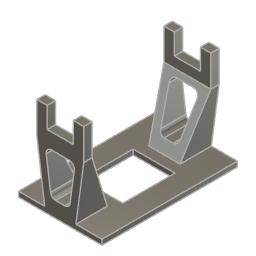
jack_stands_R (Autodesk Fusion 360 design; units mm, degrees)
Autodesk Fusion 360 part; units mm, degrees
note: some values were not read from the file. Set by a fixed rule: which sketch regions a step uses.
sketch "Esquisse1" plane through (0, 0, 0) normal (0, 0, 1) x (1, 0, 0)
  line L0 (27.5, 70) -> (52.5, 70)
  line L1 (52.5, 70) -> (52.5, 90)
  line L2 (27.5, 70) -> (27.5, 90)
  line L3 (27.5, 90) -> (17.5, 90)
  line L4 (52.5, 90) -> (62.5, 90)
  line L5 (62.5, 90) -> (62.5, 60)
  line L6 (17.5, 90) -> (17.5, 60)
  line L7 (17.5, 60) -> (25, 5)
  line L8 (25, 5) -> (0, 5)
  line L9 (0, 5) -> (0, 0)
  line L10 (0, 0) -> (80, 0)
  line L11 (80, 0) -> (80, 5)
  line L12 (80, 5) -> (55, 5)
  line L13 (55, 5) -> (62.5, 60)
  dimension "d1" = 70
  dimension "d2" = 25
  dimension "d3" = 20
  dimension "d4" = 10
  dimension "d5" = 30
  dimension "d8" = 5
  dimension "d10" = 10
  dimension "d27" = 80
  dimension "d28" = 45
  dimension "d29" = 17.5
  dimension "d30" = 30
  constraint horizontal L0
  constraint perpendicular L0 L1
  constraint perpendicular L0 L2
  constraint perpendicular L2 L3
  constraint perpendicular L1 L4
  constraint perpendicular L4 L5
  constraint equal L3 L4
  constraint perpendicular L3 L6
  constraint perpendicular L6 L8
  constraint coincident L9.end L10.start
  constraint perpendicular L8 L9
  constraint perpendicular L9 L10
  constraint perpendicular L10 L11
  constraint perpendicular L9 L12
  constraint horizontal L5.end L6.end
  constraint equal L8 L12
  constraint collinear L8 L12
  measures "d1" distance of L9.end L0
  measures "d2" distance of L0.start L0.end
  measures "d3" distance of L0.end L1.end
  measures "d4" distance of L2.end L3.end
  measures "d5" distance of L3.end L6.end
  measures "d8" distance of L8 L10
  measures "d10" vertical distance of L0.end L5.end
  measures "d27" distance of L9.end L10.end
  measures "d28" distance of L5 L6
  measures "d29" distance of L5 L11
  measures "d30" distance of L7.end L12.end
extrude "Extrusion1" add sketch "Esquisse1" along normal blind 130
sketch "Esquisse2" plane through (62.5, 0, 0) normal (1, 0, 0) x (0, 0, -1)
  line L0 (0, 60) -> (0, 90)
  line L1 (0, 90) -> (-130, 90)
  line L2 (-130, 90) -> (-130, 60)
  line L3 (-130, 60) -> (0, 60)
  line L4 (-65, 90) -> (-65, -26) construction
  line L5 (-122, 90) -> (-122, 60)
  line L6 (-122, 60) -> (-100, 5)
  line L7 (-8, 90) -> (-8, 60)
  line L8 (-8, 60) -> (-30, 5)
  line L9 (-100, 5) -> (-30, 5)
  point P0 (-130, 5)
  point P1 (0, 5)
  dimension "d13" = 8
  dimension "d14" = 30
  dimension "d15" = 30
  dimension "d16" = 8
  constraint midpoint L1 L4.start
  constraint perpendicular L1 L4
  constraint coincident L1 L5.start
  constraint coincident L3 L5.end
  constraint perpendicular L3 L5
  constraint horizontal L6.end P0
  constraint coincident L1 L7.start
  constraint coincident L3 L7.end
  constraint perpendicular L3 L7
  constraint horizontal L6.end L8.end
  measures "d13" distance of L2 L5
  measures "d14" distance of L6.end P0
  measures "d15" distance of L8.end P1
  measures "d16" distance of L0.end L7.start
extrude "Extrusion2" cut sketch "Esquisse2" against normal blind 60 contours L3 L6 L8 L9 | L1 L3 L5 L7
sketch "Esquisse3" plane through (0, 0, 130) normal (0, 0, 1) x (1, 0, 0)
  line L0 (27.5, 70) -> (27.5, 90)
  line L1 (27.5, 90) -> (17.5, 90)
  line L2 (17.5, 90) -> (17.5, 60)
  line L3 (17.5, 60) -> (25, 5)
  line L4 (25, 5) -> (0, 5)
  line L5 (0, 5) -> (0, 0)
  line L6 (0, 0) -> (80, 0)
  line L7 (80, 0) -> (80, 5)
  line L8 (80, 5) -> (55, 5)
  line L9 (55, 5) -> (62.5, 60)
  line L10 (62.5, 60) -> (62.5, 90)
  line L11 (62.5, 90) -> (52.5, 90)
  line L12 (52.5, 90) -> (52.5, 70)
  line L13 (52.5, 70) -> (27.5, 70)
  line L14 (26.5252, 49.3244) -> (30.6161, 19.3244)
  line L15 (35.5702, 15) -> (44.4298, 15)
  line L16 (49.3839, 19.3244) -> (53.4748, 49.3244)
  line L17 (48.5207, 55) -> (31.4793, 55)
  arc A0 (31.4793, 55) -> (26.5252, 49.3244) centre (31.4793, 50) ccw
  arc A1 (53.4748, 49.3244) -> (48.5207, 55) centre (48.5207, 50) ccw
  arc A2 (30.6161, 19.3244) -> (35.5702, 15) centre (35.5702, 20) ccw
  arc A3 (44.4298, 15) -> (49.3839, 19.3244) centre (44.4298, 20) ccw
  dimension "d19" = 15
  dimension "d20" = 15
  dimension "d21" = 7.5
  dimension "d22" = 7.5
  dimension "d25" = 5
  constraint horizontal L15
  constraint parallel L15 L17
  constraint parallel L3 L14
  constraint parallel L9 L16
  constraint tangent L14 A0
  constraint tangent L17 A0
  constraint tangent L16 A1
  constraint tangent L17 A1
  constraint equal A0 A1
  constraint tangent L14 A2
  constraint tangent L15 A2
  constraint equal A0 A2
  constraint tangent L15 A3
  constraint tangent L16 A3
  constraint equal A0 A3
  measures "d19" distance of L6 L15
  measures "d20" distance of L13 L17
  measures "d21" distance of L9 L16
  measures "d22" distance of L3 L14
  measures "d25" radius of A0
extrude "Extrusion3" cut sketch "Esquisse3" against normal blind 150 contours L14 L15 L16 L17 A0 A1 A2 A3
sketch "Esquisse4" plane through (0, 5, 0) normal (0, 1, 0) x (-1, 0, 0)
  line L0 (-55, 100) -> (-55, 130)
  line L1 (-55, 130) -> (-80, 130)
  line L2 (-80, 130) -> (-80, 0)
  line L3 (-80, 0) -> (-55, 0)
  line L4 (-55, 0) -> (-55, 30)
  line L5 (-55, 30) -> (-25, 30)
  line L6 (-25, 30) -> (-25, 0)
  line L7 (-25, 0) -> (0, 0)
  line L8 (0, 0) -> (0, 130)
  line L9 (0, 130) -> (-25, 130)
  line L10 (-25, 130) -> (-25, 100)
  line L11 (-25, 100) -> (-55, 100)
  line L12 (-60, 90) -> (-20, 90)
  line L13 (-20, 90) -> (-20, 40)
  line L14 (-20, 40) -> (-60, 40)
  line L15 (-60, 40) -> (-60, 90)
  constraint horizontal L12
  constraint vertical L13
  constraint horizontal L14
  constraint vertical L15
extrude "Extrusion4" cut sketch "Esquisse4" against normal blind 20 contours L12 L13 L14 L15
equation "d15 = d14"
equation "d16 = d13"
equation "d29 = ( d27 - d28 ) / 2"
